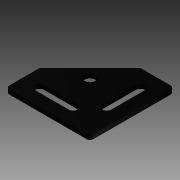
# Autodesk Inventor part: frame_gusset
Saved by Autodesk Inventor 2014 (Build 180170000, 170)
## iProperties
Created: 2013-07-15
Part Number: frame_gusset
Material: Steel, Mild
Document SubType Name: Modeling
Designer: Edward
Density: 7.86 g/cm^3
Appearance: Smooth - Black
Author: Edward
Autodesk Inventor part; units mm, degrees
ref_plane "YZ Plane" through (0, 0, 0) normal (1, 0, 0) x (0, 1, 0)
ref_plane "XZ Plane" through (0, 0, 0) normal (0, 1, 0) x (-1, 0, 0)
ref_plane "XY Plane" through (0, 0, 0) normal (0, 0, 1) x (1, 0, 0)
sketch "Sketch1" plane through (0, 0, 0) normal (0, 0, 1) x (1, 0, 0)
  line L0 (-25, -25) -> (25, -25)
  line L1 (25, -25) -> (25, 25)
  line L2 (25, 25) -> (5, 25)
  line L3 (-25, -25) -> (-25, -5)
  line L4 (-25, -5) -> (5, 25)
  point P0 (0, 0)
  dimension "d0" = 50
  dimension "d1" = 50
  dimension "d2" = 20
  dimension "d3" = 20
  dimension "d21" = 25
  dimension "d22" = 25
  constraints: 10 end point, 2 perpendicular, 1 horizontal, 1 parallel
  measures "d0" distance of L0.start L0.end
  measures "d1" distance of L0.end L1.end
  measures "d2" distance of L1.end L2.end
  measures "d3" distance of L0.start L3.end
  measures "d21" distance from line of L0 point (0, 0)
  measures "d22" distance from line of L1 point (0, 0)
extrude "Extrusion1" add sketch "Sketch1" along normal blind 2.6568
sketch "Sketch2" plane through (0, 0, 2.6568) normal (0, 0, 1) x (1, 0, 0)
  line L0 (-25, -25) -> (25, -25) projected
  line L1 (25, -25) -> (25, 25) projected
  line L2 (-15, -15) -> (5, -15) construction
  line L3 (-15, -17.75) -> (5, -17.75)
  line L4 (5, -12.25) -> (-15, -12.25)
  arc A0 (-15, -12.25) -> (-15, -17.75) centre (-15, -15) ccw
  arc A1 (5, -17.75) -> (5, -12.25) centre (5, -15) ccw
  line L5 (15, -5) -> (15, 15) construction
  line L6 (17.75, -5) -> (17.75, 15)
  line L7 (12.25, 15) -> (12.25, -5)
  arc A2 (12.25, -5) -> (17.75, -5) centre (15, -5) ccw
  arc A3 (17.75, 15) -> (12.25, 15) centre (15, 15) ccw
  point P0 (0, 0)
  point P1 (-5, -15)
  point P2 (15, 5)
  dimension "d6" = 20
  dimension "d7" = 5.5
  dimension "d8" = 10
  dimension "d9" = 20
  dimension "d10" = 20
  dimension "d11" = 5.5
  dimension "d12" = 10
  dimension "d13" = 20
  constraints: 16 end point, 8 point on circle, 8 tangent, 4 centre point, 4 parallel, 2 midpoint
  measures "d6" distance of L2.start L2.end
  measures "d7" diameter of A1
  measures "d8" distance from line of L0 L2.start
  measures "d9" distance from line of L1 L2.end
  measures "d10" distance of L5.start L5.end
  measures "d11" diameter of A3
  measures "d12" distance from line of L1 L5.start
  measures "d13" distance from line of L0 L5.start
extrude "Extrusion2" cut sketch "Sketch2" against normal through all
sketch "Sketch3" plane through (0, 0, 2.6568) normal (0, 0, 1) x (1, 0, 0)
  line L0 (-25, -25) -> (25, -25) projected
  line L1 (25, -25) -> (25, 25) projected
  circle A0 centre (-5, 5) radius 3.302
  point P0 (0, 0)
  dimension "d16" = 6.604
  dimension "d17" = 30
  dimension "d18" = 30
  constraints: 1 centre point
  measures "d16" diameter of A0
  measures "d17" distance from line of L0 A0.centre
  measures "d18" distance from line of L1 A0.centre
extrude "Extrusion3" cut sketch "Sketch3" against normal through all
fillet "Fillet1" radius 2 5 edges at (-25, -25, 1.3284) (25, -25, 1.3284) (25, 25, 1.3284) (5, 25, 1.3284) (-25, -5, 1.3284)
equation "\"d0\" = d1"
equation "\"d21\" = 0.5 * d1"
equation "\"d22\" = 0.5 * d0"
body "Solid1"
